Autodesk Inventor part; units mm, degrees
(part 2 of 2)
  spline S280 degree 2 poles (-11.9651, 36.4874) (-10.4162, 36.4874) (-8.0208, 35.5868) (-7.1383, 34.6323) knots 0 0 0 1 2 2 2
  spline S281 degree 2 poles (-7.1383, 34.6323) (-6.2378, 33.6777) (-5.2832, 30.9221) (-5.2832, 28.9229) knots 0 0 0 1 2 2 2
  line L226 (-5.2832, 28.9229) -> (-5.2832, 27.3921)
  line L227 (-5.2832, 27.3921) -> (-16.828, 27.3921)
  spline S282 degree 2 poles (-16.828, 27.3921) (-16.828, 24.4924) (-13.9103, 21.4126) (-11.3168, 21.4126) knots 0 0 0 1 2 2 2
  spline S283 degree 2 poles (-11.3168, 21.4126) (-10.3982, 21.4126) (-8.6152, 21.8268) (-7.8948, 22.151) knots 0 0 0 1 2 2 2
  spline S284 degree 2 poles (-7.8948, 22.151) (-7.1383, 22.5112) (-6.0937, 23.1416) (-5.7515, 23.4297) knots 0 0 0 1 2 2 2
  line L228 (-5.7515, 23.4297) -> (-5.5894, 23.4297)
  line L229 (-5.5894, 23.4297) -> (-5.5894, 20.3679)
  spline S285 degree 2 poles (-5.5894, 20.3679) (-6.0757, 20.1698) (-7.5526, 19.5935) (-8.1289, 19.4314) knots 0 0 0 1 2 2 2
  spline S286 degree 2 poles (-8.1289, 19.4314) (-8.9394, 19.1973) (-10.2722, 18.9631) (-11.2807, 18.9631) knots 0 0 0 1 2 2 2
  spline S287 degree 2 poles (-8.0208, 29.5353) (-8.0569, 30.67) (-8.5251, 32.3269) (-8.9754, 32.8853) knots 0 0 0 1 2 2 2
  spline S288 degree 2 poles (-8.9754, 32.8853) (-9.4617, 33.5156) (-10.9926, 34.182) (-12.1272, 34.182) knots 0 0 0 1 2 2 2
  spline S289 degree 2 poles (-12.1272, 34.182) (-13.2439, 34.182) (-14.8108, 33.5156) (-15.4592, 32.8673) knots 0 0 0 1 2 2 2
  spline S290 degree 2 poles (-15.4592, 32.8673) (-16.0896, 32.2009) (-16.7379, 30.5979) (-16.828, 29.5353) knots 0 0 0 1 2 2 2
  line L230 (-16.828, 29.5353) -> (-8.0208, 29.5353)
  line L231 (10.6561, 19.3413) -> (7.8464, 19.3413)
  line L232 (7.8464, 19.3413) -> (7.8464, 28.8509)
  spline S291 degree 2 poles (7.8464, 28.8509) (7.8464, 30.0036) (7.6303, 31.9847) (7.3061, 32.5791) knots 0 0 0 1 2 2 2
  spline S292 degree 2 poles (7.3061, 32.5791) (6.9639, 33.2095) (5.7392, 33.8218) (4.6946, 33.8218) knots 0 0 0 1 2 2 2
  spline S293 degree 2 poles (4.6946, 33.8218) (3.65, 33.8218) (1.4347, 32.7052) (0.3721, 31.8046) knots 0 0 0 1 2 2 2
  line L233 (0.3721, 31.8046) -> (0.3721, 19.3413)
  line L234 (0.3721, 19.3413) -> (-2.4376, 19.3413)
  line L235 (-2.4376, 19.3413) -> (-2.4376, 36.0191)
  line L236 (-2.4376, 36.0191) -> (0.3721, 36.0191)
  line L237 (0.3721, 36.0191) -> (0.3721, 34.164)
  spline S294 degree 2 poles (0.3721, 34.164) (1.6328, 35.2987) (4.0642, 36.4874) (5.433, 36.4874) knots 0 0 0 1 2 2 2
  spline S295 degree 2 poles (5.433, 36.4874) (7.8825, 36.4874) (10.6561, 33.2455) (10.6561, 30.1657) knots 0 0 0 1 2 2 2
  line L238 (10.6561, 30.1657) -> (10.6561, 19.3413)
  line L239 (17.4641, 19.3413) -> (14.6544, 19.3413)
  line L240 (14.6544, 19.3413) -> (14.6544, 36.0191)
  line L241 (14.6544, 36.0191) -> (17.4641, 36.0191)
  line L242 (17.4641, 36.0191) -> (17.4641, 19.3413)
  line L243 (17.6622, 38.7927) -> (14.4743, 38.7927)
  line L244 (14.4743, 38.7927) -> (14.4743, 41.7104)
  line L245 (14.4743, 41.7104) -> (17.6622, 41.7104)
  line L246 (17.6622, 41.7104) -> (17.6622, 38.7927)
  line L247 (34.6821, 19.3413) -> (31.8725, 19.3413)
  line L248 (31.8725, 19.3413) -> (31.8725, 28.8509)
  spline S296 degree 2 poles (31.8725, 28.8509) (31.8725, 30.0036) (31.6564, 31.9847) (31.3322, 32.5791) knots 0 0 0 1 2 2 2
  spline S297 degree 2 poles (31.3322, 32.5791) (30.99, 33.2095) (29.7653, 33.8218) (28.7207, 33.8218) knots 0 0 0 1 2 2 2
  spline S298 degree 2 poles (28.7207, 33.8218) (27.676, 33.8218) (25.4607, 32.7052) (24.3981, 31.8046) knots 0 0 0 1 2 2 2
  line L249 (24.3981, 31.8046) -> (24.3981, 19.3413)
  line L250 (24.3981, 19.3413) -> (21.5885, 19.3413)
  line L251 (21.5885, 19.3413) -> (21.5885, 36.0191)
  line L252 (21.5885, 36.0191) -> (24.3981, 36.0191)
  line L253 (24.3981, 36.0191) -> (24.3981, 34.164)
  spline S299 degree 2 poles (24.3981, 34.164) (25.6589, 35.2987) (28.0903, 36.4874) (29.4591, 36.4874) knots 0 0 0 1 2 2 2
  spline S300 degree 2 poles (29.4591, 36.4874) (31.9085, 36.4874) (34.6821, 33.2455) (34.6821, 30.1657) knots 0 0 0 1 2 2 2
  line L254 (34.6821, 30.1657) -> (34.6821, 19.3413)
  spline S301 degree 2 poles (39.2208, 16.6758) (39.509, 16.5497) (40.6076, 16.1535) (41.31, 15.9914) knots 0 0 0 1 2 2 2
  spline S302 degree 2 poles (41.31, 15.9914) (42.0845, 15.7933) (43.3992, 15.5591) (44.1737, 15.5591) knots 0 0 0 1 2 2 2
  spline S303 degree 2 poles (44.1737, 15.5591) (45.4705, 15.5591) (47.2715, 16.2435) (47.7758, 16.8559) knots 0 0 0 1 2 2 2
  spline S304 degree 2 poles (47.7758, 16.8559) (48.2621, 17.4682) (48.6403, 19.0712) (48.6403, 20.0978) knots 0 0 0 1 2 2 2
  line L255 (48.6403, 20.0978) -> (48.6403, 21.5566)
  spline S305 degree 2 poles (48.6403, 21.5566) (47.5056, 20.5661) (45.3264, 19.6295) (43.6874, 19.6295) knots 0 0 0 1 2 2 2
  spline S306 degree 2 poles (43.6874, 19.6295) (40.8417, 19.6295) (37.4738, 23.862) (37.4738, 27.8423) knots 0 0 0 1 2 2 2
  spline S307 degree 2 poles (37.4738, 27.8423) (37.4738, 29.9135) (38.6445, 33.1194) (39.617, 34.2541) knots 0 0 0 1 2 2 2
  spline S308 degree 2 poles (39.617, 34.2541) (40.5536, 35.3167) (43.1291, 36.4874) (44.4979, 36.4874) knots 0 0 0 1 2 2 2
  spline S309 degree 2 poles (44.4979, 36.4874) (45.7946, 36.4874) (47.6858, 35.875) (48.6403, 35.3167) knots 0 0 0 1 2 2 2
  line L256 (48.6403, 35.3167) -> (48.8024, 36.0191)
  line L257 (48.8024, 36.0191) -> (51.45, 36.0191)
  line L258 (51.45, 36.0191) -> (51.45, 21.2505)
  spline S310 degree 2 poles (51.45, 21.2505) (51.45, 17) (47.7578, 13.0377) (43.9576, 13.0377) knots 0 0 0 1 2 2 2
  spline S311 degree 2 poles (43.9576, 13.0377) (42.7329, 13.0377) (40.1754, 13.4339) (39.0767, 13.7581) knots 0 0 0 1 2 2 2
  line L259 (39.0767, 13.7581) -> (39.0767, 16.6758)
  line L260 (39.0767, 16.6758) -> (39.2208, 16.6758)
  line L261 (48.6403, 23.862) -> (48.6403, 33.0294)
  spline S312 degree 2 poles (48.6403, 33.0294) (47.5957, 33.5336) (45.8307, 33.9659) (44.9481, 33.9659) knots 0 0 0 1 2 2 2
  spline S313 degree 2 poles (44.9481, 33.9659) (42.8229, 33.9659) (40.3735, 30.8321) (40.3735, 27.8963) knots 0 0 0 1 2 2 2
  spline S314 degree 2 poles (40.3735, 27.8963) (40.3735, 25.1227) (42.2286, 22.223) (44.3178, 22.223) knots 0 0 0 1 2 2 2
  spline S315 degree 2 poles (44.3178, 22.223) (45.4164, 22.223) (47.7218, 23.0875) (48.6403, 23.862) knots 0 0 0 1 2 2 2
  point P0 (0, 0)
  dimension "d6" = 25.4
  constraints: 2 end point, 2 horizontal, 4 other
  measures "d6" distance between parallel lines of L4 L2
emboss "Emboss1" sketch "Sketch3" operation cut depth 2.54 direction (0, 0, -1) wrap yes faces at (75.1505, 135.4667, 34.1601) (42.5763, 135.4667, 70.7231) (-75.0162, 135.4667, 34.454) contours S154 S155 L0 S158 S159 | L0 S159 S160 S157 S158 S155 S156 S153 S154 | S215 S207 S208 S209 L1 S216 S217 S218 S219 L174 L171 S211 S212 | L1 S212 S213 L172 L173 S214 S215 | S38 S39 S40 S41 L0 S46 S47 | L0 S47 S48 S49 L58 L59 L60 L61 L62 S50 S51 S38 | L1 L174 S216 S209 S210 L170 L171 | L0 S41 S42 S43 L56 L57 S44 S45 S46 | S152 S136 L105 L106 S137 S138 S139 L1 | L1 S139 S140 S141 S149 S150 S151 S152 | S141 S142 S143 S144 S145 L1 S146 S147 S148 S149 | S145 L107 L108 S146 L1 | S0 S1 S2 S3 S4 S5 L5 L6 S6 S7 S8 S9 S10 S11 S12 S13 L7 L8 S14 S15 | L9 L10 L11 L12 L13 L14 L15 L16 | S16 S17 L20 L21 L22 S18 S19 S20 S21 L23 L24 L25 S22 S23 | L26 L27 L28 L29 L30 L31 L32 L33 | L34 L35 L36 L37 L38 L39 L40 L41 L42 L43 L44 L45 | S24 S25 S26 S27 S28 S29 S30 S31 | L46 L47 L48 L49 L50 L51 L52 L53 L54 L55 | S52 S53 S54 S55 S56 S57 L63 S58 S59 S60 L64 L65 S61 S62 S63 L66 L67 L68 | S68 L70 L71 L72 L73 L74 L75 L76 L77 L78 L79 L80 S69 S70 S71 L81 L82 S72 | S73 S74 S75 S76 L83 L84 S77 S78 S79 L85 L86 S80 S81 | S86 S87 S88 S89 S90 L88 L89 S91 S92 S93 S94 S95 L90 L91 S96 S97 | L92 L93 L94 L95 | S98 S99 S100 S101 | S106 L96 L97 S107 S108 S109 S110 S111 S112 S113 S114 S115 L98 L99 S116 S117 S118 S119 S120 S121 S122 | S123 S124 S125 S126 L100 L101 S127 S128 S129 L102 L103 S130 S131 | L109 L110 S161 S162 S163 L111 L112 L113 L114 L115 S164 S165 L116 | S166 S167 S168 S169 L117 L118 S170 S171 S172 L119 L120 S173 S174 | L122 S179 S180 S181 S182 L123 L124 L125 S183 S184 S185 L126 L127 L128 L129 L130 S186 S187 S188 S189 S190 L131 L132 | L133 L134 L135 L136 | L137 L138 L139 L140 | L141 L142 S191 S192 S193 L143 L144 L145 L146 L147 S194 S195 L148 | L149 L150 S196 S197 S198 L151 L152 L153 S199 S200 S201 L154 L155 L156 | S202 L157 L158 L159 L160 L161 L162 L163 L164 L165 L166 L167 S203 S204 S205 L168 L169 S206 | S220 S221 S222 S223 S224 S225 L175 S226 S227 S228 L176 L177 S229 S230 S231 L178 L179 L180 | L182 S236 S237 L183 L184 L185 L186 L187 L188 L189 L190 L191 L192 L193 S238 S239 L194 | S240 L195 L196 L197 L198 L199 L200 L201 L202 L203 L204 L205 S241 S242 S243 L206 L207 S244 | S245 S246 S247 S248 L208 L209 S249 S250 S251 L210 L211 S252 S253 | L213 S258 S259 L214 L215 L216 L217 L218 S260 S261 L219 | S262 S263 S264 S265 | S270 S271 L220 L221 L222 L223 L224 S272 S273 | S278 S279 S280 S281 L226 L227 S282 S283 S284 L228 L229 S285 S286 | L231 L232 S291 S292 S293 L233 L234 L235 L236 L237 S294 S295 L238 | L239 L240 L241 L242 | L243 L244 L245 L246 | L247 L248 S296 S297 S298 L249 L250 L251 L252 L253 S299 S300 L254 | S301 S302 S303 S304 L255 S305 S306 S307 S308 S309 L256 L257 L258 S310 S311 L259 L260
body "Solid1"
